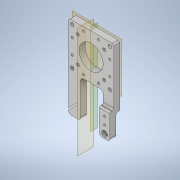
# Autodesk Inventor part: 30_XY_Sample_lightsheetarm_v3
Saved by Autodesk Inventor 2022 (Build 260153000, 153)
## iProperties
Created: 2020-12-29
Part Number: 30_XY_Sample_lightsheetarm_v3
Material: Generic
Document SubType Name: Modeling
Designer: diederichbenedict
Density: 1 g/cm^3
Appearance: Default
Author: diederichbenedict
Autodesk Inventor part; units mm, degrees
ref_plane "YZ Plane" through (0, 0, 0) normal (1, 0, 0) x (0, 1, 0)
ref_plane "XZ Plane" through (0, 0, 0) normal (0, 1, 0) x (-1, 0, 0)
ref_plane "XY Plane" through (0, 0, 0) normal (0, 0, 1) x (1, 0, 0)
ref_plane "Work Plane1" through (0, 0, 0) normal (0, 0, 1) x (1, 0, 0)
sketch "Sketch1" plane through (0, 0, 0) normal (0, 0, 1) x (1, 0, 0)
  circle A0 centre (-10, -25) radius 1.45 projected
  circle A1 centre (-10, 25) radius 1.45 projected
  circle A2 centre (10, 25) radius 1.45 projected
  circle A3 centre (10, -25) radius 1.45 projected
  circle A4 centre (-25, 25) radius 2.325 projected
  circle A5 centre (25, -25) radius 2.325 projected
  circle A6 centre (-25, -25) radius 2.325 projected
  circle A7 centre (25, 25) radius 2.325 projected
  line L0 (28, 30) -> (30, 28) projected
  line L1 (28, 30) -> (-28, 30) projected
  line L2 (-30, 28) -> (-28, 30) projected
  line L3 (-30, 28) -> (-30, -28) projected
  line L4 (-28, -30) -> (-30, -28) projected
  line L5 (-28, -30) -> (28, -30) projected
  line L6 (30, -28) -> (28, -30) projected
  line L7 (30, -28) -> (30, 28) projected
  circle A8 centre (-17.5, -17.5) radius 1.95 projected
  circle A9 centre (17.5, 17.5) radius 1.95 projected
  circle A10 centre (17.5, -17.5) radius 1.95 projected
  circle A11 centre (-17.5, 17.5) radius 1.95 projected
  circle A12 centre (0, 0) radius 7.5 projected
  circle A13 centre (-25.33, -75.26) radius 6.15 projected
  circle A14 centre (25, -10) radius 1.45 projected
  circle A15 centre (-25, -10) radius 1.45 projected
  circle A16 centre (-25, 10) radius 1.45 projected
  circle A17 centre (25, 10) radius 1.45 projected
  point P0 (0, 0)
extrude "Extrusion1" add sketch "Sketch1" along normal blind 8 contours L0 L7 L6 L5 L4 L3 L2 L1
sketch "Sketch2" plane through (0, 0, 8) normal (0, 0, 1) x (1, 0, 0)
  circle A0 centre (0, 0) radius 7.5 projected
  circle A1 centre (25, 10) radius 1.45 projected
  circle A2 centre (-25, 10) radius 1.45 projected
  circle A3 centre (-25, -10) radius 1.45 projected
  circle A4 centre (25, -10) radius 1.45 projected
  circle A5 centre (10, -25) radius 1.45 projected
  circle A6 centre (10, 25) radius 1.45 projected
  circle A7 centre (-10, 25) radius 1.45 projected
  circle A8 centre (-10, -25) radius 1.45 projected
  line L0 (-28, -30) -> (28, -30) projected
  line L1 (28, -30) -> (30, -28) projected
  line L2 (30, -28) -> (30, 28) projected
  line L3 (30, 28) -> (28, 30) projected
  line L4 (28, 30) -> (-28, 30) projected
  line L5 (30, -28) -> (30, 28) projected
  line L6 (30, -30) -> (16, -30)
  line L7 (16, -30) -> (16, -80)
  line L8 (16, -80) -> (30, -80)
  line L9 (30, -80) -> (30, -30)
  line L10 (30, 28) -> (30, -28) projected
  line L11 (30, -30) -> (30, -28)
  line L12 (30, -28) -> (28, -30)
  line L13 (-28, 30) -> (-30, 28) projected
  line L14 (-30, 28) -> (-30, -28) projected
  line L15 (-30, -28) -> (-28, -30) projected
  line L16 (-30, -30) -> (-14, -30)
  line L17 (-14, -30) -> (-14, -80)
  line L18 (-14, -80) -> (-30, -80)
  line L19 (-30, -80) -> (-30, -30)
  line L20 (-30, -30) -> (-30, -28)
  line L21 (-30, -28) -> (-28, -30)
  line L22 (-28, -30) -> (-30, -30)
  line L23 (28, -30) -> (30, -28) projected
  line L24 (28, -30) -> (30, -30)
  line L25 (30, -30) -> (30, -28)
  line L26 (30, -28) -> (28, -30)
  circle A9 centre (-17.5, 17.5) radius 1.95 projected
  circle A10 centre (-25, 25) radius 2.325 projected
  circle A11 centre (25, 25) radius 2.325 projected
  circle A12 centre (17.5, 17.5) radius 1.95 projected
  circle A13 centre (17.5, -17.5) radius 1.95 projected
  circle A14 centre (25, -25) radius 2.325 projected
  circle A15 centre (-25, -25) radius 2.325 projected
  point P0 (0, 0)
  point P1 (-24.2387, -104)
  dimension "d57" = 14
  dimension "d58" = 50
  dimension "d59" = 16
  constraints: 32 end point, 5 point on line, 4 parallel, 3 collinear, 3 perpendicular, 2 horizontal, 2 vertical
  measures "d57" distance of L8.end L7.end
  measures "d58" distance of L7.end L6.end
  measures "d59" distance of L17.end L18.end
extrude "Extrusion2" add sketch "Sketch2" against normal up to surface (8 mm away) contours L16 L20 L15 | L0 L17 L18 L19 L16 | L0 L6 L9 L8 L7 | L1 L11 L6
fillet "Fillet1" radius 4 6 edges at (30, -80, 4) (16, -80, 4) (-14, -80, 4) (-30, -80, 4) (-14, -30, 4) (16, -30, 4)
ref_plane "Work Plane2" through (-6, -91, 19) normal (1, 0, 0) x (0, 0, -1)
sketch "Sketch8" plane through (0, 0, 8) normal (0, 0, 1) x (1, 0, 0)
  circle A0 centre (0, 0) radius 16
  point P0 (0, 0)
  dimension "d41" = 32
  constraints: 1 centre point, 1 coincident
  measures "d41" diameter of A0
extrude "Extrusion7" cut sketch "Sketch8" against normal through all
sketch "Sketch11" plane through (0, 0, 8) normal (0, 0, 1) x (1, 0, 0)
  circle A0 centre (0, 0) radius 16 projected
  circle A1 centre (25, 25) radius 2.325 projected
  circle A2 centre (-25, -25) radius 2.325 projected
  circle A3 centre (25, -25) radius 2.325 projected
  circle A4 centre (-25, 25) radius 2.325 projected
  circle A5 centre (-17.5, 17.5) radius 1.95 projected
  circle A6 centre (17.5, -17.5) radius 1.95 projected
  circle A7 centre (17.5, 17.5) radius 1.95 projected
  circle A8 centre (-17.5, -17.5) radius 1.95 projected
  circle A9 centre (25, 10) radius 1.45 projected
  circle A10 centre (-25, 10) radius 1.45 projected
  circle A11 centre (-25, -10) radius 1.45 projected
  circle A12 centre (25, -10) radius 1.45 projected
  circle A13 centre (10, -25) radius 1.45 projected
  circle A14 centre (10, 25) radius 1.45 projected
  circle A15 centre (-10, 25) radius 1.45 projected
  circle A16 centre (-10, -25) radius 1.45 projected
  arc A17 (16, -76) -> (20, -80) centre (20, -76) ccw projected
  line L0 (20, -80) -> (26, -80) projected
  arc A18 (26, -80) -> (30, -76) centre (26, -76) ccw projected
  line L1 (30, 28) -> (30, -76) projected
  line L2 (30, 28) -> (28, 30) projected
  line L3 (28, 30) -> (-28, 30) projected
  line L4 (-28, 30) -> (-30, 28) projected
  line L5 (-10, -30) -> (12, -30) projected
  arc A19 (16, -34) -> (12, -30) centre (12, -34) ccw projected
  line L6 (16, -34) -> (16, -76) projected
  circle A20 centre (23, -74) radius 3.75
  circle A21 centre (23, -64) radius 1.45
  circle A22 centre (23, -54) radius 1.45
  arc A23 (-30, -76) -> (-26, -80) centre (-26, -76) ccw projected
  line L7 (-18, -80) -> (-26, -80) projected
  arc A24 (-18, -80) -> (-14, -76) centre (-18, -76) ccw projected
  line L8 (-14, -34) -> (-14, -76) projected
  arc A25 (-10, -30) -> (-14, -34) centre (-10, -34) ccw projected
  line L9 (-30, 28) -> (-30, -76) projected
  point P0 (0, 0)
  dimension "d77" = 7.5
  dimension "d80" = 2.9
  dimension "d81" = 2.9
  dimension "d82" = 10
  dimension "d83" = 10
  dimension "d84" = 6
  constraints: 3 centre point
  measures "d77" diameter of A20
  measures "d80" diameter of A21
  measures "d81" diameter of A22
  measures "d82" distance of A21.centre A20.centre
  measures "d83" distance of A22.centre A21.centre
  measures "d84" distance from line of L0 A20.centre
extrude "Extrusion10" cut sketch "Sketch11" against normal through all contours A20 | A21 | A22
sketch "Sketch12" plane through (16, -76, 8) normal (-1, 0, 0) x (0, 0, 1)
  line L0 (-8, -1.75) -> (-8, 5.75) projected
  line L1 (0, 5.75) -> (0, -1.75) projected
  circle A0 centre (-4.3852, 2) radius 1.45
  point P0 (-8, 76)
  dimension "d85" = 2.9
  constraints: 1 centre point
  measures "d85" diameter of A0
extrude "Extrusion11" cut sketch "Sketch12" against normal through all
sketch "Sketch13" plane through (0, 0, 8) normal (0, 0, 1) x (1, 0, 0)
  circle A0 centre (23, -54) radius 1.45 projected
  circle A1 centre (23, -64) radius 1.45 projected
  circle A2 centre (23, -74) radius 3.75 projected
  circle A3 centre (0, 0) radius 16 projected
  arc A4 (-30, -76) -> (-26, -80) centre (-26, -76) ccw projected
  line L0 (-30, -76) -> (-30, 28) projected
  line L1 (-30, 28) -> (-28, 30) projected
  line L2 (-28, 30) -> (28, 30) projected
  line L3 (28, 30) -> (30, 28) projected
  line L4 (30, 28) -> (30, -76) projected
  arc A5 (26, -80) -> (30, -76) centre (26, -76) ccw projected
  line L5 (26, -80) -> (20, -80) projected
  arc A6 (16, -76) -> (20, -80) centre (20, -76) ccw projected
  line L6 (16, -76) -> (16, -34) projected
  arc A7 (16, -34) -> (12, -30) centre (12, -34) ccw projected
  line L7 (12, -30) -> (-10, -30) projected
  arc A8 (-10, -30) -> (-14, -34) centre (-10, -34) ccw projected
  line L8 (-14, -34) -> (-14, -76) projected
  arc A9 (-18, -80) -> (-14, -76) centre (-18, -76) ccw projected
  line L9 (-18, -80) -> (-26, -80) projected
  circle A10 centre (25, 25) radius 2.325 projected
  circle A11 centre (-25, -25) radius 2.325 projected
  circle A12 centre (25, -25) radius 2.325 projected
  circle A13 centre (-25, 25) radius 2.325 projected
  circle A14 centre (-17.5, 17.5) radius 1.95 projected
  circle A15 centre (17.5, -17.5) radius 1.95 projected
  circle A16 centre (17.5, 17.5) radius 1.95 projected
  circle A17 centre (-17.5, -17.5) radius 1.95 projected
  circle A18 centre (25, 10) radius 1.45 projected
  circle A19 centre (-25, 10) radius 1.45 projected
  circle A20 centre (-25, -10) radius 1.45 projected
  circle A21 centre (25, -10) radius 1.45 projected
  circle A22 centre (10, -25) radius 1.45 projected
  circle A23 centre (10, 25) radius 1.45 projected
  circle A24 centre (-10, 25) radius 1.45 projected
  circle A25 centre (-10, -25) radius 1.45 projected
  line L10 (-36.3192, -79.6068) -> (-18.6416, -61.9292)
  line L11 (-18.6416, -61.9292) -> (-17.5809, -62.9898)
  line L12 (-17.5809, -62.9898) -> (-35.2586, -80.6675)
  line L13 (-35.2586, -80.6675) -> (-36.3192, -79.6068)
  line L14 (-36.3192, -79.6068) -> (-17.5809, -62.9898) construction
  line L15 (-18.6416, -61.9292) -> (-35.2586, -80.6675) construction
  line L16 (-36.3192, -79.6068) -> (-11.3192, -79.6068) construction
  point P0 (0, 0)
  point P1 (-26.9501, -71.2983)
  dimension "d88" = 25
  dimension "d89" = 45
  dimension "d90" = 1.5
  constraints: 14 end point, 2 midpoint, 2 parallel, 1 equal length, 1 horizontal, 1 perpendicular
  measures "d88" distance of L10.start L10.end
  measures "d89" angle of L16 L10
  measures "d90" distance of L10.end L11.end
extrude "Extrusion12" cut sketch "Sketch13" against normal blind 10 contours L12 L13 L10 L0 | L0 L10 L11 L12
sketch "Sketch14" plane through (-15.0607, -58.3483, 8) normal (-0.7071068, 0.7071068, 0) x (-0.7071068, -0.7071068, 0)
  line L0 (22.6274, -8) -> (5.0642, -8) projected
  line L1 (5.0642, 0) -> (22.6274, 0) projected
  line L2 (5.0642, 0) -> (5.0642, -8) projected
  circle A0 centre (18.1437, -4) radius 1.45
  circle A1 centre (10.5109, -4) radius 1.45
  line L3 (22.6274, 0) -> (22.6274, -8) projected
  point P0 (-51.9079, -8)
  dimension "d93" = 2.9
  dimension "d94" = 2.9
  constraints: 2 centre point
  measures "d93" diameter of A0
  measures "d94" diameter of A1
extrude "Extrusion13" cut sketch "Sketch14" along normal through all contours A0 | A1
ref_plane "Work Plane3" through (0, 28, 0) normal (-1, 0, 0) x (0, 0, 1)
sketch "Sketch15" plane through (0, 0, 8) normal (0, 0, 1) x (1, 0, 0)
  line L0 (-30, -73.2876) -> (-18.6416, -61.9292) construction
  line L1 (-18.6416, -61.9292) -> (-17.5809, -62.9898) construction
  line L2 (-17.5809, -62.9898) -> (-30, -75.4089) construction
  line L3 (-30, -75.4089) -> (-30, -76) construction
  arc A0 (-30, -76) -> (-26, -80) centre (-26, -76) ccw construction
  line L4 (-18, -80) -> (-26, -80) construction
  arc A1 (-18, -80) -> (-14, -76) centre (-18, -76) ccw construction
  line L5 (-14, -34) -> (-14, -76) construction
  arc A2 (-10, -30) -> (-14, -34) centre (-10, -34) ccw construction
  line L6 (-10, -30) -> (12, -30) construction
  arc A3 (16, -34) -> (12, -30) centre (12, -34) ccw construction
  line L7 (16, -34) -> (16, -76) projected
  arc A4 (16, -76) -> (20, -80) centre (20, -76) ccw projected
  line L8 (20, -80) -> (26, -80) projected
  arc A5 (26, -80) -> (30, -76) centre (26, -76) ccw projected
  line L9 (30, 28) -> (30, -76) projected
  line L10 (30, 28) -> (28, 30) construction
  line L11 (28, 30) -> (-28, 30) construction
  line L12 (-28, 30) -> (-30, 28) construction
  line L13 (-30, 28) -> (-30, -73.2876) construction
  circle A6 centre (-10, -25) radius 1.45 construction
  circle A7 centre (-10, 25) radius 1.45 construction
  circle A8 centre (10, 25) radius 1.45 construction
  circle A9 centre (10, -25) radius 1.45 construction
  circle A10 centre (25, -10) radius 1.45 construction
  circle A11 centre (-25, -10) radius 1.45 construction
  circle A12 centre (-25, 10) radius 1.45 construction
  circle A13 centre (25, 10) radius 1.45 construction
  circle A14 centre (-17.5, -17.5) radius 1.95 construction
  circle A15 centre (17.5, 17.5) radius 1.95 construction
  circle A16 centre (17.5, -17.5) radius 1.95 construction
  circle A17 centre (-17.5, 17.5) radius 1.95 construction
  circle A18 centre (-25, 25) radius 2.325 construction
  circle A19 centre (25, -25) radius 2.325 construction
  circle A20 centre (-25, -25) radius 2.325 construction
  circle A21 centre (25, 25) radius 2.325 construction
  circle A22 centre (0, 0) radius 16 construction
  circle A23 centre (23, -74) radius 3.75 projected
  circle A24 centre (23, -64) radius 1.45 projected
  circle A25 centre (23, -54) radius 1.45 projected
  line L14 (16, -76) -> (16, -34) construction
  line L15 (16, -45.7691) -> (30, -45.7691)
  point P0 (0, 0)
  constraints: 2 end point, 2 point on line, 1 horizontal
extrude "Extrusion14" add sketch "Sketch15" along normal blind 5
sketch "Sketch16" plane through (0, 0, 0) normal (0, 0, -1) x (-1, 0, 0)
  line L0 (-30, -76) -> (-30, -45.7691) projected
  line L1 (-30, -45.7691) -> (-16, -45.7691) construction
  line L2 (-16, -45.7691) -> (-16, -76) projected
  arc A0 (-20, -80) -> (-16, -76) centre (-20, -76) ccw projected
  line L3 (-20, -80) -> (-26, -80) projected
  arc A1 (-30, -76) -> (-26, -80) centre (-26, -76) ccw projected
  circle A2 centre (-23, -74) radius 3.75 projected
  circle A3 centre (-23, -54) radius 1.45 projected
  circle A4 centre (-23, -64) radius 1.45 projected
  line L4 (-30, -50.7691) -> (-16, -50.7691)
  line L5 (-16, -76) -> (-16, -34) construction
  point P0 (0, 0)
  dimension "d99" = 5
  constraints: 2 end point, 2 point on line, 1 horizontal
  measures "d99" distance between parallel lines of L1 L4
extrude "Extrusion15" cut sketch "Sketch16" against normal blind 5
fillet "Fillet2" radius 2 4 edges at (23, -50.7691, 0) (23, -45.7691, 13) (23, -45.7691, 8) (23, -50.7691, 5)
sketch "Sketch17" plane through (20, -80, 13) normal (0, -1, 0) x (1, 0, 0)
  line L0 (0, -8) -> (6, -8) projected
  line L1 (6, 0) -> (6, -8) projected
  line L2 (0, 0) -> (6, 0) projected
  line L3 (0, -8) -> (0, 0) projected
  circle A0 centre (3, -4) radius 1.4
  point P0 (-20, -13)
  dimension "d103" = 2.8
  constraints: 1 centre point
  measures "d103" diameter of A0
extrude "Extrusion16" cut sketch "Sketch17" against normal blind 10 contours A0
body "Solid1"
